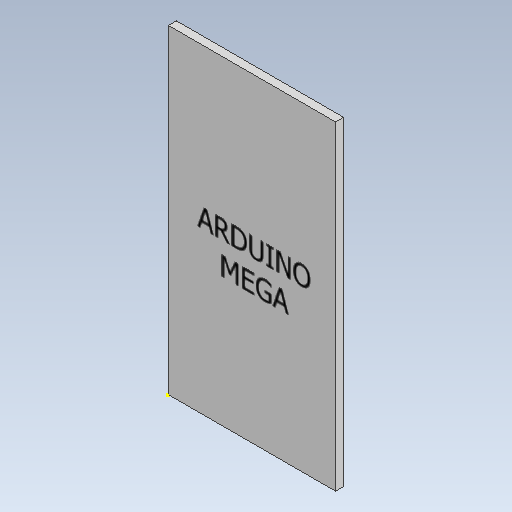
# Autodesk Inventor part: mega_sketch
Saved by Autodesk Inventor 2020 (Build 240168000, 168)
## iProperties
Created: 2019-10-23
Part Number: mega_sketch
Material: Generic
Document SubType Name: Modeling
Designer: Connor
Density: 1 g/cm^3
Appearance: Default
Author: Connor
Autodesk Inventor part; units mm, degrees
ref_plane "YZ Plane" through (0, 0, 0) normal (1, 0, 0) x (0, 1, 0)
ref_plane "XZ Plane" through (0, 0, 0) normal (0, 1, 0) x (-1, 0, 0)
ref_plane "XY Plane" through (0, 0, 0) normal (0, 0, 1) x (1, 0, 0)
sketch "Sketch1" plane through (0, 0, 0) normal (0, 0, 1) x (1, 0, 0)
  line L0 (0, 0) -> (0, 101.6)
  line L1 (0, 101.6) -> (53.086, 101.6)
  line L2 (53.086, 101.6) -> (53.086, 0)
  line L3 (53.086, 0) -> (0, 0)
  dimension "d0" = 101.6
  dimension "d1" = 53.086
  constraints: 8 end point, 3 perpendicular, 1 vertical
  measures "d0" distance of L0.start L0.end
  measures "d1" distance of L0.end L1.end
extrude "Extrusion1" add sketch "Sketch1" along normal blind 2.54
sketch "Sketch2" plane through (0, 0, 2.54) normal (0, 0, 1) x (1, 0, 0)
  line L0 (8.9572, 57.2265) -> (45.6416, 57.2265) construction
  line L1 (45.6416, 57.2265) -> (45.6416, 22.0966) construction
  line L2 (45.6416, 22.0966) -> (8.9572, 22.0966) construction
  line L3 (8.9572, 22.0966) -> (8.9572, 57.2265) construction
  point P0 (0, 0)
  constraints: 2 other
body "Solid1"
